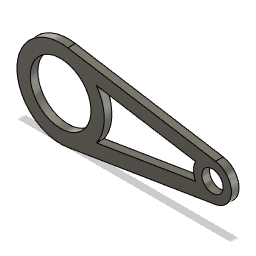
Shoppingcart_key_cnc (Autodesk Fusion 360 design; units mm, degrees)
Autodesk Fusion 360 part; units mm, degrees
sketch "Skizze1" plane through (0, 0, 0) normal (0, 0, 1) x (1, 0, 0)
  circle A0 centre (0, 0) radius 11.5
  circle A1 centre (40, 0) radius 5
  line L0 (1.8687, 11.3471) -> (40.8125, 4.9335)
  line L1 (40.8125, -4.9335) -> (1.8687, -11.3471)
  circle A2 centre (40, 0) radius 2.8
  circle A3 centre (0, 0) radius 8
  line L2 (9.4516, 6.5512) -> (35.5375, 2.2551)
  line L3 (9.4516, -6.5512) -> (35.5375, -2.2551)
  dimension "d1" = 23
  dimension "d2" = 10
  dimension "d3" = 40
  dimension "d6" = 2.2
  dimension "d7" = 3.5
  constraint coincident A0.centre A3.centre
  constraint horizontal A0.centre A1.centre
  constraint coincident A0 L0.start
  constraint coincident A1 L0.end
  constraint coincident A1 L1.start
  constraint coincident A0 L1.end
  constraint tangent A0 L1
  constraint tangent A0 L0
  constraint tangent A1 L0
  constraint tangent A1 L1
  constraint concentric A1 A2
  constraint concentric A0 A3
  constraint coincident A0 L2.start
  constraint coincident A1 L2.end
  constraint coincident A0 L3.start
  constraint coincident A1 L3.end
  constraint parallel L0 L2
  constraint parallel L1 L3
  constraint tangent A3 L2
  constraint tangent A3 L3
  measures "d1" diameter of A0
  measures "d2" diameter of A1
  measures "d3" distance of A0.centre A1.centre
  measures "d6" distance of A1 A2
  measures "d7" distance of A0 A3
extrude "Extrusion1" add sketch "Skizze1" along normal blind 2 contours A0 | A0 A1 L0 L2 | A0 A1 L1 L3 | A1
